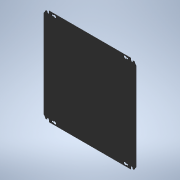
# Autodesk Inventor part: 166X_02_00_P6_(2)
Saved by Autodesk Inventor 2021 (Build 250183000, 183)
## iProperties
Created: 2025-09-22
Part Number: 166X_02_00_P6_(2)
Material: Generic
Catalog Web Link: www.cadenas.de
Description: AE 2.0 Montageplatte-AE 2.0 Montageplatte
Vendor: RITTAL
Document SubType Name: Modeling
Designer: psAdmin
Manufacturer: RITTAL
Mass: 783.312 g
Surface Area: 6331.1 cm^2
Volume: 783.312 cm^3
Density: 1 g/cm^3
Appearance: PSOLRGB-176-176-176
Category: PARTsolutions
Company: RITTAL
Title: 166X_02_00_P6
Author: Cadenas PARTsolutions
Comments: AE 2.0 Montageplatte
PSOL_IDENT_0: {$CADENAS_DATA/23d-libs/rittal/schaltschranksys/kompakt_schaltschr/parts_ae_2_0/montageplatte_ae_2_0
PSOL_IDENT_1: .prj},197 {VTYP=3D},{NB=166X_02_00_P6_(2)},{LINA=166X_02_00_P6},{NN=AE 2.0 Montageplatte},{DATE=28.0
PSOL_IDENT_2: 4.2025 21:11:32},{GEOMDATE=11.04.2025 07:46:14},{VERSION=},{LINEID=350},{WBVAR=DETAIL},{WBNUMERIC=DE
PSOL_IDENT_3: TAIL}  {NB=166X_02_00_P6_(2)},{LINA=166X_02_00_P6},{KT=DUMMY},{BEST=166X},{B=600},{H=600},{S=2.5},{T=
PSOL_IDENT_4: MIN},{B1=550},{H1=575},{VERS=3},{DETAIL=2},{BEZ1=Neues Kompaktgehäuse},{BEZ2=Stahlblech},{BEZ3=eintü
PSOL_IDENT_5: rig},{F=550},{G=575},{CNSECLASS51=27-18-01-02},{CNSECLASS70=27-18-01-01},{CNSECLASS80=27-18-01-01},{
PSOL_IDENT_6: CNSETIM40=EC000261}
NB: 166X_02_00_P6_(2)
NN: AE 2.0 Montageplatte
NT: AE 2.0 Montageplatte
NBSYN: $BEST._02_00_P6_($DETAIL.)
LINA: 166X_02_00_P6
CATALOG: Rittal
BEST: 166X
B: 600
H: 600
S: 2.5
T: 0
B1: 550
H1: 575
VERS: 3
DETAIL: niedrig
BEZ1: Neues Kompaktgehäuse
BEZ2: Stahlblech
BEZ3: eintürig
F: 550
G: 575
CNSECLASS70: 27-18-01-01
CNSECLASS80: 27-18-01-01
SUPPLIER: RITTAL
ARTICLENO: 166X_02_00_P6_(2)
BOMINFO: 166X_02_00_P6
CREATOR: CADENAS GmbH
Autodesk Inventor part; units mm, degrees
sketch "Sketch_12" plane through (0, 0, 0) normal (0, 0, 1) x (1, 0, 0)
  line L0 (-275, 538.5) -> (-275, 11.5)
  line L1 (-275, 11.5) -> (-273.5, 11.5)
  line L2 (-273.5, 11.5) -> (-263.9737, -5)
  line L3 (-263.9737, -5) -> (-255.5, -5)
  line L4 (-255.5, -5) -> (-255.5, 0)
  arc A0 (-244.5, 0) -> (-255.5, 0) centre (-250, 0) ccw
  line L5 (-244.5, 0) -> (-244.5, -12.5)
  line L6 (-244.5, -12.5) -> (244.5, -12.5)
  line L7 (244.5, -12.5) -> (244.5, 0)
  arc A1 (255.5, 0) -> (244.5, 0) centre (250, 0) ccw
  line L8 (255.5, 0) -> (255.5, -5)
  line L9 (255.5, -5) -> (263.9737, -5)
  line L10 (263.9737, -5) -> (273.5, 11.5)
  line L11 (273.5, 11.5) -> (275, 11.5)
  line L12 (275, 11.5) -> (275, 538.5)
  line L13 (275, 538.5) -> (273.5, 538.5)
  line L14 (273.5, 538.5) -> (263.9737, 555)
  line L15 (263.9737, 555) -> (255.5, 555)
  line L16 (255.5, 555) -> (255.5, 550)
  arc A2 (244.5, 550) -> (255.5, 550) centre (250, 550) ccw
  line L17 (244.5, 550) -> (244.5, 562.5)
  line L18 (244.5, 562.5) -> (-244.5, 562.5)
  line L19 (-244.5, 562.5) -> (-244.5, 550)
  arc A3 (-255.5, 550) -> (-244.5, 550) centre (-250, 550) ccw
  line L20 (-255.5, 550) -> (-255.5, 555)
  line L21 (-255.5, 555) -> (-263.9737, 555)
  line L22 (-263.9737, 555) -> (-273.5, 538.5)
  line L23 (-273.5, 538.5) -> (-275, 538.5)
  arc A4 (216.8088, 4.2) -> (216.8088, -4.2) centre (210, 0) ccw
  line L24 (216.8088, -4.2) -> (229, -4.2)
  line L25 (229, -4.2) -> (229, 4.2)
  line L26 (229, 4.2) -> (216.8088, 4.2)
  arc A5 (216.8088, 554.2) -> (216.8088, 545.8) centre (210, 550) ccw
  line L27 (216.8088, 545.8) -> (229, 545.8)
  line L28 (229, 545.8) -> (229, 554.2)
  line L29 (229, 554.2) -> (216.8088, 554.2)
  line L30 (-229, 4.2) -> (-229, -4.2)
  line L31 (-229, -4.2) -> (-216.8088, -4.2)
  arc A6 (-216.8088, -4.2) -> (-216.8088, 4.2) centre (-210, 0) ccw
  line L32 (-216.8088, 4.2) -> (-229, 4.2)
  line L33 (-229, 554.2) -> (-229, 545.8)
  line L34 (-229, 545.8) -> (-216.8088, 545.8)
  arc A7 (-216.8088, 545.8) -> (-216.8088, 554.2) centre (-210, 550) ccw
  line L35 (-216.8088, 554.2) -> (-229, 554.2)
  constraints: 72 end point, 16 point on circle, 8 centre point
extrude "Extrusion1" add sketch "Sketch_12" against normal blind 2.5
ref_plane "MP_XY" through (0, 0, 0) normal (0, 0, 1) x (1, 0, 0)
ref_plane "MP_YZ" through (0, 0, 0) normal (1, 0, 0) x (0, 1, 0)
ref_plane "MP_ZX" through (0, 0, 0) normal (0, 1, 0) x (0, 0, 1)
ref_plane "to_EB_XY" through (224.8, 0, -2.5) normal (0, 0, 1) x (1, 0, 0)
ref_plane "to_EB_YZ" through (224.8, 0, -2.5) normal (1, 0, 0) x (0, 1, 0)
ref_plane "to_EB_ZX" through (224.8, 0, -2.5) normal (0, 1, 0) x (0, 0, 1)
body "Solid1"
